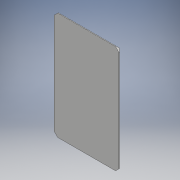
# Autodesk Inventor part: Деталь1
Saved by Autodesk Inventor 2018.1 (Build 221171000, 171)
## iProperties
Created: 2023-03-15
Part Number: Деталь1
Material: Типовые
Document SubType Name: Modeling
Designer: Student
Density: 1 g/cm^3
Appearance: По умолчанию
Author: Student
Autodesk Inventor part; units mm, degrees
ref_plane "YZ Plane" through (0, 0, 0) normal (1, 0, 0) x (0, 1, 0)
ref_plane "XZ Plane" through (0, 0, 0) normal (0, 1, 0) x (-1, 0, 0)
ref_plane "XY Plane" through (0, 0, 0) normal (0, 0, 1) x (1, 0, 0)
sketch "Эскиз1" plane through (0, 0, 0) normal (0, 1, 0) x (-1, 0, 0)
  line L0 (57.0205, 86.1427) -> (-37.9795, 86.1427)
  line L1 (-37.9795, 86.1427) -> (-37.9795, -71.8573)
  line L2 (-37.9795, -71.8573) -> (57.0205, -71.8573)
  line L3 (57.0205, -71.8573) -> (57.0205, 86.1427)
  point P0 (0, 0)
  dimension "d0" = 158
  dimension "d1" = 95
  constraints: 8 end point, 2 parallel, 1 horizontal, 1 perpendicular
  measures "d0" distance of L2.end L0.start
  measures "d1" distance of L1.end L2.end
extrude "Выдавливание1" add sketch "Эскиз1" along normal blind 10
chamfer "Фаска1" distance 9 angle 45 1 edges at (-9.5205, 10, 86.1427) measured on face at (-25.3538, 3.3333, 86.1427)
chamfer "Фаска2" distance 9 angle 45 1 edges at (37.9795, 10, 2.6427) measured on face at (6.3129, 10, 27.476)
chamfer "Фаска3" distance 9 angle 45 1 edges at (-57.0205, 10, 2.6427) measured on face at (-57.0205, 3.3333, 30.476)
chamfer "Фаска4" distance 9 angle 45 1 edges at (-9.5205, 10, -71.8573) measured on face at (-22.3538, 3.3333, -71.8573)
chamfer "Фаска5" distance 5 angle 45 1 edges at (-57.0205, 0.5, -71.8573) measured on face at (-25.3538, 0.3333, -71.8573)
chamfer "Фаска6" distance 5 angle 45 1 edges at (-57.0205, 0.5, 86.1427) measured on face at (-57.0205, 0.3333, -15.8573)
chamfer "Фаска7" distance 5 angle 45 1 edges at (37.9795, 0.5, -71.8573) measured on face at (37.9795, 0.6667, -19.1907)
chamfer "Фаска8" distance 5 angle 45 1 edges at (37.9795, 0.5, 86.1427) measured on face at (37.9795, 0.6667, -15.8573)
